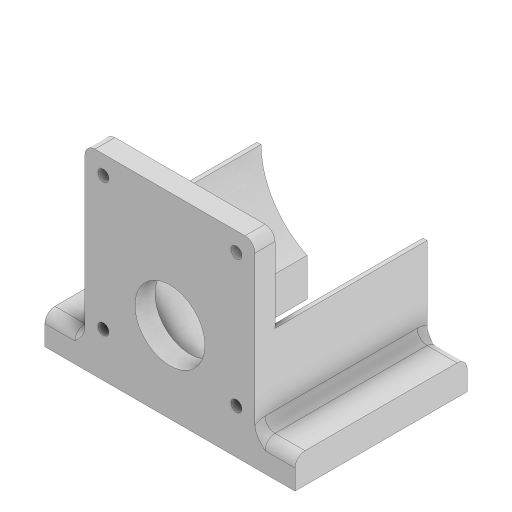
# Autodesk Inventor part: PIEZA_JACLUBER
Saved by Autodesk Inventor 2024.3 (Build 283343000, 343)
## iProperties
Created: 2024-06-21
Part Number: PIEZA_JACLUBER
Material: Generic
Document SubType Name: Modeling
Designer: Niler
Density: 1 g/cm^3
Appearance: Default
Author: Niler
Autodesk Inventor part; units mm, degrees
ref_plane "YZ Plane" through (0, 0, 0) normal (1, 0, 0) x (0, 1, 0)
ref_plane "XZ Plane" through (0, 0, 0) normal (0, 1, 0) x (-1, 0, 0)
ref_plane "XY Plane" through (0, 0, 0) normal (0, 0, 1) x (1, 0, 0)
sketch "Sketch1" plane through (0, 0, 0) normal (0, 0, 1) x (1, 0, 0)
  line L0 (-33.234, 33.234) -> (33.234, -33.234) construction
  line L1 (33.234, 33.234) -> (-33.234, -33.234) construction
  circle A0 centre (0, 0) radius 47
  line L2 (-33.234, -33.234) -> (33.234, 33.234)
  line L3 (-33.234, 33.234) -> (33.234, -33.234)
  circle A1 centre (-33.234, 33.234) radius 2.75
  circle A2 centre (33.234, 33.234) radius 2.75
  circle A3 centre (33.234, -33.234) radius 2.75
  circle A4 centre (-33.234, -33.234) radius 2.75
  line L4 (-42.5, 42.5) -> (42.5, 42.5)
  line L5 (42.5, 42.5) -> (42.5, -42.5)
  line L6 (42.5, -42.5) -> (-42.5, -42.5)
  line L7 (-42.5, -42.5) -> (-42.5, 42.5)
  line L8 (-42.5, 42.5) -> (42.5, -42.5) construction
  line L9 (42.5, 42.5) -> (-42.5, -42.5) construction
  dimension "d2" = 94
  dimension "d3" = 5.5
  dimension "d4" = 5.5
  dimension "d5" = 5.5
  dimension "d6" = 5.5
  dimension "d14" = 85
  dimension "d15" = 85
  constraints: 20 end point, 5 centre point, 5 coincident, 4 midpoint, 4 point on circle, 2 parallel, 1 horizontal, 1 perpendicular
  measures "d2" diameter of A0
  measures "d3" diameter of A1
  measures "d4" diameter of A2
  measures "d5" diameter of A3
  measures "d6" diameter of A4
  measures "d14" distance of L5.end L6.end
  measures "d15" distance of L4.end L5.end
extrude "Extrusion1" add sketch "Sketch1" along normal blind 10 contours L5 A0 A3 L3 L2 A2 | A0 A2 L4 L5 | L5 L6 A0 A3 | L2 L3 A1 A0 L4 A2 | A3 A0 L6 A4 L2 L3 | L2 A4 A0 L7 A1 L3 | A0 A1 L7 L4 | L6 L7 A0 A4
sketch "Sketch2" plane through (0, 0, 10) normal (0, 0, 1) x (1, 0, 0)
  line L0 (0, 0) -> (0, -15)
  circle A0 centre (0, -15) radius 5
  circle A1 centre (0, -15) radius 17.5
  dimension "d9" = 15
  dimension "d10" = 10
  dimension "d11" = 35
  constraints: 2 centre point, 2 coincident, 2 end point, 1 vertical
  measures "d9" distance of L0.start L0.end
  measures "d10" diameter of A0
  measures "d11" diameter of A1
extrude "Extrusion2" cut sketch "Sketch2" against normal blind 10 contours A0 | A1
sketch "Sketch3" plane through (0, 0, 0) normal (0, 0, -1) x (-1, 0, 0)
  circle A0 centre (0, 0) radius 40.5
  line L0 (-42.5, 55.5) -> (42.5, 55.5)
  line L1 (42.5, 55.5) -> (42.5, -55.5)
  line L2 (42.5, -55.5) -> (-42.5, -55.5)
  line L3 (-42.5, -55.5) -> (-42.5, 55.5)
  line L4 (-42.5, 55.5) -> (42.5, -55.5) construction
  line L5 (42.5, 55.5) -> (-42.5, -55.5) construction
  line L6 (-42.5, -42.5) -> (-42.5, 42.5) projected
  line L7 (-42.5, 0) -> (42.5, 0)
  point P0 (40.5, 0)
  point P1 (-40.5, 0)
  point P2 (40.5, 0)
  point P3 (-40.5, 0)
  dimension "d16" = 81
  dimension "d17" = 85
  dimension "d18" = 111
  constraints: 14 end point, 4 midpoint, 2 parallel, 1 centre point, 1 coincident, 1 horizontal, 1 perpendicular
  measures "d16" diameter of A0
  measures "d17" distance of L1.end L2.end
  measures "d18" distance of L0.end L1.end
extrude "Extrusion3" add sketch "Sketch3" along normal blind 76 contours L7 L1 L2 L3 A0
sketch "Sketch4" plane through (-42.5, -42.5, 10) normal (0, -1, 0) x (1, 0, 0)
  line L0 (0, -10) -> (85, -10) projected
  line L1 (85, -10) -> (85, 0) projected
  line L2 (0, 0) -> (85, 0) projected
  line L3 (0, -10) -> (0, 0) projected
  point P0 (42.5, -10)
extrude "Extrusion4" add sketch "Sketch4" along normal blind 13
sketch "Sketch5" plane through (42.5, 42.5, 10) normal (1, 0, 0) x (0, 0, -1)
  line L0 (0, -98) -> (86, -98) projected
  line L1 (0, -98) -> (86, -98)
  line L2 (86, -98) -> (86, -83)
  line L3 (86, -83) -> (0, -83)
  line L4 (0, -83) -> (0, -98)
  point P0 (10, -42.5)
  dimension "d23" = 86
  dimension "d24" = 15
  constraints: 8 end point, 2 parallel, 1 horizontal, 1 perpendicular
  measures "d23" distance of L3.end L2.end
  measures "d24" distance of L2.end L1.end
extrude "Extrusion5" add sketch "Sketch5" along normal blind 20
mirror "Mirror1" about plane through (0, 0, 0) normal (1, 0, 0) of "Extrusion5"
fillet "Fillet1" radius 5 8 edges at (42.5, -40.5, -33) (-52.5, -40.5, -76) (-42.5, -40.5, -33) (-52.5, -40.5, 10) (52.5, -40.5, -76) (52.5, -40.5, 10) (42.5, 42.5, 5) (-42.5, 42.5, 5)
sketch "Sketch6" plane through (0, 0, -76) normal (0, 0, -1) x (-1, 0, 0)
  line L0 (-17.5, 70) -> (17.5, 70)
  line L1 (17.5, 70) -> (17.5, -70)
  line L2 (17.5, -70) -> (-17.5, -70)
  line L3 (-17.5, -70) -> (-17.5, 70)
  line L4 (-17.5, 70) -> (17.5, -70) construction
  line L5 (17.5, 70) -> (-17.5, -70) construction
  point P0 (0, 0)
  dimension "d28" = 35
  dimension "d29" = 140
  constraints: 12 end point, 2 midpoint, 2 parallel, 1 horizontal, 1 perpendicular
  measures "d28" distance of L1.end L2.end
  measures "d29" distance of L0.end L1.end
extrude "Extrusion6" cut sketch "Sketch6" against normal blind 40
fillet "Fillet2" radius 10 2 edges at (-17.5, -46.012, -36) (17.5, -46.012, -36)
sketch "Sketch7" plane through (47.5, -40.5, 5) normal (0, 1, 0) x (1, 0, 0)
  point P0 (-47.5, 5)
body "Solid1"
